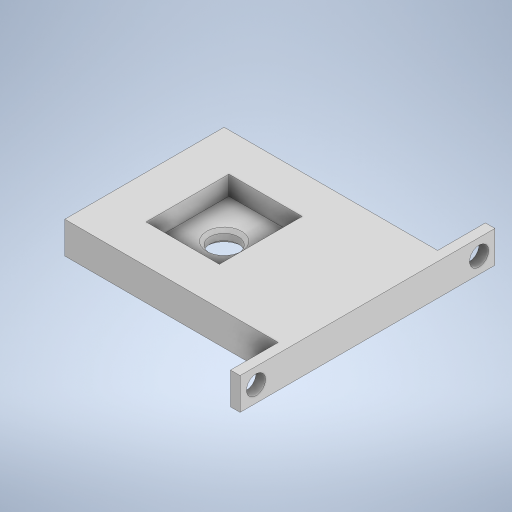
# Autodesk Inventor part: Стенка энкодер
Saved by Autodesk Inventor 2023 (Build 270158000, 158)
## iProperties
Created: 2022-05-02
Part Number: Стенка энкодер
Material: Типовые
Document SubType Name: Modeling
Designer: User
Density: 1 g/cm^3
Appearance: По умолчанию
Author: User
Autodesk Inventor part; units mm, degrees
ref_plane "YZ Plane" through (0, 0, 0) normal (1, 0, 0) x (0, 1, 0)
ref_plane "XZ Plane" through (0, 0, 0) normal (0, 1, 0) x (-1, 0, 0)
ref_plane "XY Plane" through (0, 0, 0) normal (0, 0, 1) x (1, 0, 0)
sketch "Эскиз1" plane through (0, 0, 0) normal (0, 1, 0) x (-1, 0, 0)
  line L0 (0, 0) -> (-70, 0)
  line L1 (-70, 0) -> (-70, -50)
  line L2 (-70, -50) -> (0, -50)
  line L3 (0, -50) -> (0, 0)
  line L4 (-70, 0) -> (-25, 0)
  line L5 (-25, 0) -> (-25, -25)
  line L6 (-25, -25) -> (-70, -25)
  line L7 (-70, -25) -> (-70, 0)
  circle A0 centre (-25, -25) radius 4.5
  line L8 (-70, -50) -> (-70, -65)
  line L9 (-70, -65) -> (-67, -65)
  line L10 (-67, -65) -> (-67, -50)
  line L11 (-70, 0) -> (-70, 15)
  line L12 (-70, 15) -> (-67, 15)
  line L13 (-67, 15) -> (-67, 0)
  point P0 (-67, 0)
  dimension "d0" = 70
  dimension "d1" = 50
  dimension "d2" = 45
  dimension "d3" = 25
  dimension "d4" = 9
  dimension "d31" = 15
  dimension "d32" = 3
  dimension "d33" = 15
  dimension "d34" = 3
  constraints: 28 end point, 5 point on line, 4 parallel, 4 perpendicular, 2 horizontal, 1 centre point, 1 coincident, 1 vertical
  measures "d0" distance of L2.end L1.end
  measures "d1" distance of L1.end L0.end
  measures "d2" distance of L5.end L6.end
  measures "d3" distance of L4.end L5.end
  measures "d4" diameter of A0
  measures "d31" distance of L1.end L8.end
  measures "d32" distance of L8.end L9.end
  measures "d33" distance of L0.end L11.end
  measures "d34" distance of L11.end L12.end
extrude "Выдавливание1" add sketch "Эскиз1" along normal blind 4 contours L3 L2 L1 L6 A0 L5 L0 | L5 A0 L6 L1 L0 | L0 L11 L12 L13 | L10 L9 L8 L2
sketch "Эскиз2" plane through (0, 4, 0) normal (0, 1, 0) x (1, 0, 0)
  circle A0 centre (25, 25) radius 4.5 projected
  line L0 (25, 25) -> (25, 12)
  line L1 (25, 12) -> (13.5, 12)
  line L2 (13.5, 12) -> (36.5, 12)
  line L3 (36.5, 12) -> (36.5, 38)
  line L4 (36.5, 38) -> (13.5, 38)
  line L5 (13.5, 38) -> (13.5, 12)
  line L6 (67, 50) -> (0, 50) projected
  line L7 (0, 0) -> (70, 0)
  line L8 (70, 0) -> (70, 50)
  line L9 (70, 50) -> (0, 50)
  line L10 (0, 50) -> (0, 0)
  line L11 (70, -15) -> (70, 65) projected
  line L12 (67, 65) -> (67, 50) projected
  line L13 (70, 65) -> (67, 65)
  line L14 (67, 65) -> (67, 50)
  line L15 (67, 50) -> (70, 50)
  line L16 (70, 50) -> (70, 65)
  line L17 (67, -15) -> (70, -15) projected
  line L18 (67, 0) -> (67, -15) projected
  line L19 (70, -15) -> (67, -15)
  line L20 (67, -15) -> (67, 0)
  line L21 (67, 0) -> (70, 0)
  line L22 (70, 0) -> (70, -15)
  dimension "d7" = 13
  dimension "d8" = 11.5
  dimension "d9" = 23
  dimension "d10" = 26
  constraints: 36 end point, 8 parallel, 5 perpendicular, 4 horizontal, 1 vertical
  measures "d7" distance of L0.start L0.end
  measures "d8" distance of L0.end L1.end
  measures "d9" distance of L4.end L3.end
  measures "d10" distance of L3.end L2.end
extrude "Выдавливание2" add sketch "Эскиз2" along normal blind 6 contours L9 L8 L7 L10 L6 | L12 L13 L11 L9 | L11 L17 L18 L7
chamfer "Фаска1" distance 1 angle 45 2 edges at (29.5, 0, -25) (29.5, 4, -25)
sketch "Эскиз4" plane through (70, 0, 15) normal (1, 0, 0) x (0, 0, -1)
  line L0 (0, 0) -> (0, 10) projected
  line L1 (0, 5) -> (5, 5)
  line L2 (80, 0) -> (80, 10) projected
  line L3 (80, 5) -> (75, 5)
  circle A0 centre (5, 5) radius 3
  circle A1 centre (75, 5) radius 3
  point P0 (15, 0)
  dimension "d35" = 5
  dimension "d36" = 5
  dimension "d37" = 6
  dimension "d38" = 6
  constraints: 4 end point, 2 centre point, 2 coincident, 2 midpoint, 1 horizontal, 1 point on line
  measures "d35" distance of L1.start L1.end
  measures "d36" distance of L3.start L3.end
  measures "d37" diameter of A0
  measures "d38" diameter of A1
extrude "Выдавливание4" cut sketch "Эскиз4" against normal blind 3.75
